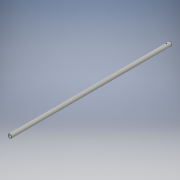
# Autodesk Inventor part: catapultArmWithSaladBowl
Saved by Autodesk Inventor 2016 SP1 (Build 200210100, 210)
## iProperties
Created: 2016-01-16
Part Number: catapultArmWithSaladBowl
Material: Generic
Document SubType Name: Modeling
Designer: steele
Density: 1 g/cm^3
Appearance: Default
Author: steele
Autodesk Inventor part; units mm, degrees
ref_plane "XY Plane" through (0, 0, 0) normal (0, 0, 1) x (1, 0, 0)
sketch "Sketch7" plane through (0, 0, 0) normal (0, 0, 1) x (1, 0, 0)
  circle A0 centre (0, 0) radius 9.525
  circle A1 centre (0, 0) radius 13.97
  dimension "d25" = 27.94
  dimension "d26" = 19.05
  constraints: 2 centre point, 2 coincident
  measures "d25" diameter of A1
  measures "d26" diameter of A0
extrude "Extrusion4" add sketch "Sketch7" along normal blind 1117.6
ref_plane "Work Plane5" through (13.97, 0, 0) normal (1, 0, 0) x (0, 1, 0)
ref_plane "Work Plane6" through (0, 13.97, 0) normal (0, 1, 0) x (-1, 0, 0)
sketch "Sketch9" plane through (0, 13.97, 0) normal (0, 1, 0) x (-1, 0, 0)
  circle A0 centre (0, 25.4) radius 3.302
  line L0 (-13.97, 0) -> (13.97, 0) projected
  point P0 (0, 0)
  dimension "d33" = 25.4
  dimension "d34" = 6.604
  constraints: 1 centre point
  measures "d33" distance from line of A0.centre L0
  measures "d34" diameter of A0
extrude "Extrusion6" cut sketch "Sketch9" against normal through all
equation "\"d25\" = ballHolderPipeOutsideDiam"
equation "\"d26\" = ballHolderPipeInsideDiam"
equation "\"d27\" = ballHolderLoopHandleLength"
equation "\"d33\" = catapulutArmSaldBoleHoleDistanceFromEnd"
equation "\"d34\" = catapultArmSaladBowlHoleDiam"
equation "\"d35\" = ballHolderLoopHandleLength"
equation "\"ballHolderLoopDiam\" = 203.2"
equation "\"ballHolderLoopHandleLength\" = 1117.6"
equation "\"xxx\" = 0.5 * ballHolderLoopDiam + ballHolderLoopHandleLength"
equation "\"ballHolderPipeInsideDiam\" = 19.05"
equation "\"ballHolderPipeOutsideDiam\" = 27.94"
equation "\"ballHolderLoopRadius\" = 0.5 * ballHolderLoopDiam"
equation "\"ballHolderAxelDiam\" = 6.604"
equation "\"ballHolderAxelDistanceFromEnd\" = 25.4"
equation "\"catapultArmSaladBowlHoleDiam\" = 6.604"
equation "\"catapulutArmSaldBoleHoleDistanceFromEnd\" = 25.4"
equation "\"ballDiam\" = 247.65"
equation "\"ballRadius\" = 0.5 * ballDiam"
equation "\"saladHolderThickness\" = 2.54"
equation "\"holeForAirCylinderDiam\" = 6.35"
equation "\"holeForAirCylinderDistanceFromEnd\" = 127"
body "Solid3"
